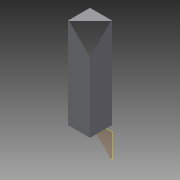
# Autodesk Inventor part: front peice right
Saved by Autodesk Inventor 2015 (Build 190159000, 159)
## iProperties
Created: 2014-10-04
Part Number: front peice right
Material: Generic
Document SubType Name: Modeling
Designer: jesse
Density: 1 g/cm^3
Appearance: Default
Author: jesse
Autodesk Inventor part; units mm, degrees
ref_plane "YZ Plane" through (0, 0, 0) normal (1, 0, 0) x (0, 1, 0)
ref_plane "XZ Plane" through (0, 0, 0) normal (0, 1, 0) x (-1, 0, 0)
ref_plane "XY Plane" through (0, 0, 0) normal (0, 0, 1) x (1, 0, 0)
ref_plane "Work Plane1" through (0, -84.7502, 0) normal (0, 0, 1) x (1, 0, 0)
sketch "Sketch1" plane through (0, -84.7502, 0) normal (0, 0, 1) x (1, 0, 0)
  line L0 (9.525, 94.2752) -> (-9.525, 94.2752) projected
  line L1 (-9.525, 15.4232) -> (9.525, 15.4232) projected
  line L2 (-9.525, 94.2752) -> (-9.525, 15.4232)
  line L3 (9.525, 15.4232) -> (9.525, 94.2752)
  point P0 (0, 84.7502)
  constraints: 4 end point, 1 perpendicular, 1 vertical
extrude "Extrusion1" add sketch "Sketch1" along normal blind 19.05
body "Solid1"
